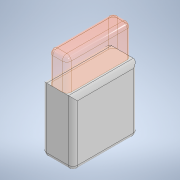
# Autodesk Inventor part: battery_1S_100mAh
Saved by Autodesk Inventor 2021 (Build 250183000, 183)
## iProperties
Created: 2022-02-27
Part Number: battery_1S_100mAh
Material: Generic
Document SubType Name: Modeling
Designer: ermoz
Density: 1 g/cm^3
Appearance: Default
Author: ermoz
Autodesk Inventor part; units mm, degrees
ref_plane "YZ Plane" through (0, 0, 0) normal (1, 0, 0) x (0, 1, 0)
ref_plane "XZ Plane" through (0, 0, 0) normal (0, 1, 0) x (-1, 0, 0)
ref_plane "XY Plane" through (0, 0, 0) normal (0, 0, 1) x (1, 0, 0)
sketch "Sketch1" plane through (0, 0, 0) normal (1, 0, 0) x (0, 1, 0)
  line L0 (0, 0) -> (14.5, 0)
  line L1 (14.5, 0) -> (14.5, -14.5)
  line L2 (14.5, -14.5) -> (0, -14.5)
  line L3 (0, -14.5) -> (0, 0)
  dimension "d5" = 14.5
  dimension "d6" = 14.5
  constraints: 8 end point, 2 parallel, 1 horizontal, 1 perpendicular
  measures "d5" distance of L1.end L2.end
  measures "d6" distance of L0.end L1.end
extrude "Extrusion1" add sketch "Sketch1" along normal blind 6.88
sketch "Sketch2" plane through (0, 14.5, 0) normal (0, 1, 0) x (1, 0, 0)
  line L0 (0, 14.5) -> (0, 0) projected
  line L1 (0, 0) -> (6.88, 0) projected
  line L2 (6.88, 14.5) -> (6.88, 0) projected
  line L3 (0, 14.5) -> (6.88, 14.5) projected
  line L4 (1.39, 0) -> (5.49, 0)
  line L5 (5.49, 0) -> (5.49, 14.5)
  line L6 (5.49, 14.5) -> (1.39, 14.5)
  line L7 (1.39, 14.5) -> (1.39, 0)
  line L8 (0, 14.5) -> (6.88, 14.5) projected
  line L9 (0, 0) -> (6.88, 0) projected
  dimension "d12" = 4.1
  dimension "d13" = 1.39
  constraints: 8 end point, 2 collinear, 2 parallel, 1 horizontal, 1 perpendicular
  measures "d12" distance between parallel lines of L5 L7
  measures "d13" distance between parallel lines of L7 L0
extrude "Extrusion2" add sketch "Sketch2" along normal blind 7 separate body contours L3 L5 L1 L7
fillet "Fillet1" radius 1 10 edges at (0, 0, -7.25) (0, 7.25, -14.5) (3.44, 0, -14.5) (6.88, 7.25, -14.5) (6.88, 0, -7.25) (6.88, 7.25, 0) (0, 7.25, 0) (3.44, 0, 0) (0, 14.5, -7.25) (6.88, 14.5, -7.25)
fillet "Fillet2" radius 1 8 edges at (1.39, 18, 0) (5.49, 18, 0) (1.39, 18, -14.5) (5.49, 18, -14.5) (1.39, 21.5, -7.25) (3.44, 21.5, 0) (5.49, 21.5, -7.25) (3.44, 21.5, -14.5)
body "Solid1"
body "Solid2"
